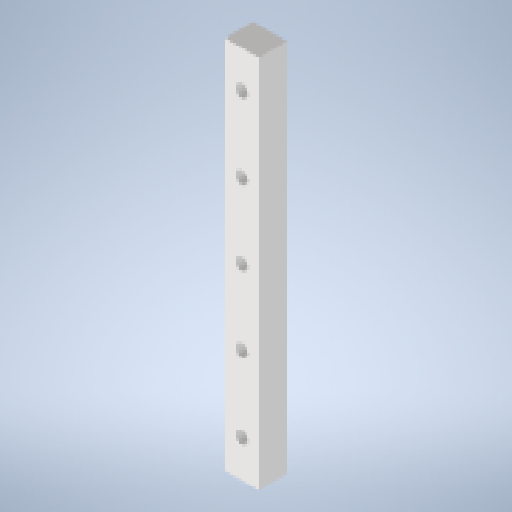
# Autodesk Inventor part: LinearRail
Saved by Autodesk Inventor 2023 (Build 270158000, 158)
## iProperties
Created: 2023-08-31
Part Number: LinearRail
Material: Steel, Carbon
Document SubType Name: Modeling
Designer: Felix
Density: 7.85 g/cm^3
Appearance: Semi-Polished
Author: Felix
Autodesk Inventor part; units mm, degrees
ref_plane "YZ Plane" through (0, 0, 0) normal (1, 0, 0) x (0, 1, 0)
ref_plane "XZ Plane" through (0, 0, 0) normal (0, 1, 0) x (-1, 0, 0)
ref_plane "XY Plane" through (0, 0, 0) normal (0, 0, 1) x (1, 0, 0)
sketch "Sketch1" plane through (0, 0, 0) normal (0, 1, 0) x (-1, 0, 0)
  line L0 (-4.5, -3.25) -> (4.5, -3.25)
  line L1 (4.5, -3.25) -> (4.5, 3.25)
  line L2 (4.5, 3.25) -> (-4.5, 3.25)
  line L3 (-4.5, 3.25) -> (-4.5, -3.25)
  line L4 (-4.5, -3.25) -> (4.5, 3.25) construction
  line L5 (4.5, -3.25) -> (-4.5, 3.25) construction
  point P0 (0, 0)
  dimension "d0" = 9
  dimension "d1" = 6.5
  constraints: 12 end point, 2 midpoint, 2 parallel, 1 horizontal, 1 perpendicular
  measures "d0" distance of L2.end L1.end
  measures "d1" distance of L1.end L0.end
extrude "Extrusion1" add sketch "Sketch1" along normal blind 100
sketch "Sketch2" plane through (4.5, 0, -3.25) normal (0, 0, -1) x (-1, 0, 0)
  line L0 (0, 0) -> (9, 0) construction
  line L1 (9, 0) -> (9, 100) construction
  line L2 (0, 100) -> (9, 100) construction
  line L3 (0, 0) -> (0, 100) construction
  line L4 (9, 100) -> (0, 100) projected
  line L5 (4.5, 100) -> (4.5, 0) construction
  point P0 (4.5, 90)
  point P1 (4.5, 70)
  point P2 (4.5, 50)
  point P3 (4.5, 30)
  point P4 (4.5, 10)
  dimension "d4" = 20
  dimension "d5" = 20
  dimension "d6" = 20
  dimension "d7" = 20
  dimension "d9" = 10
  dimension "d10" = 10
  constraints: 4 point on line, 2 end point, 2 midpoint, 1 perpendicular
  measures "d4" distance of point (4.5, 70) point (4.5, 90)
  measures "d5" distance of point (4.5, 50) point (4.5, 70)
  measures "d6" distance of point (4.5, 30) point (4.5, 50)
  measures "d7" distance of point (4.5, 10) point (4.5, 30)
  measures "d9" distance from line of point (4.5, 90) L2
  measures "d10" distance from line of point (4.5, 10) L0
hole "Hole1" at (0, 90, -3.25) at (0, 70, -3.25) at (0, 50, -3.25) at (0, 30, -3.25) at (0, 10, -3.25) direction (0, 0, 1) diameter 3.4 depth 8 counterbore diameter 6.8 counterbore depth 3.75 clearance for "Hex Head Cap Screw DIN EN 24017" size "M3" standard "DIN"
equation "\"d5\" = d4"
equation "\"d6\" = d5"
equation "\"d7\" = d4"
equation "\"d9\" = d10"
body "Solid1"
